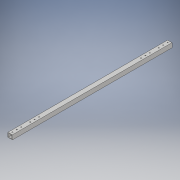
# Autodesk Inventor part: 3ft 1x1
Saved by Autodesk Inventor 2018 (Build 220112000, 112)
## iProperties
Created: 2018-12-30
Part Number: 3ft 1x1
Material: Generic
Document SubType Name: Modeling
Designer: maste
Density: 1 g/cm^3
Appearance: Default
Author: maste
Autodesk Inventor part; units mm, degrees
ref_plane "YZ Plane" through (0, 0, 0) normal (1, 0, 0) x (0, 1, 0)
ref_plane "XZ Plane" through (0, 0, 0) normal (0, 1, 0) x (-1, 0, 0)
ref_plane "XY Plane" through (0, 0, 0) normal (0, 0, 1) x (1, 0, 0)
sketch "Sketch1" plane through (0, 0, 0) normal (0, 0, 1) x (1, 0, 0)
  line L0 (0, 0) -> (25.4, 0)
  line L1 (25.4, 0) -> (25.4, 25.4)
  line L2 (25.4, 25.4) -> (0, 25.4)
  line L3 (0, 25.4) -> (0, 0)
  line L4 (3.175, 22.225) -> (22.225, 22.225)
  line L5 (22.225, 22.225) -> (22.225, 3.175)
  line L6 (22.225, 3.175) -> (3.175, 3.175)
  line L7 (3.175, 3.175) -> (3.175, 22.225)
  dimension "d0" = 25.4
  dimension "d1" = 25.4
  dimension "d2" = 3.175
  constraints: 16 end point, 4 parallel, 2 perpendicular, 1 horizontal, 3 other
  measures "d0" distance of L2.end L1.end
  measures "d1" distance of L1.end L0.end
  measures "d2" distance between parallel lines of L2 L4
extrude "Extrusion1" add sketch "Sketch1" along normal blind 914.4
sketch "Sketch2" plane through (0, 25.4, 0) normal (0, 1, 0) x (1, 0, 0)
  line L0 (0, 0) -> (25.4, 0) construction
  line L1 (12.7, 0) -> (12.7, -12.7) construction
  line L2 (12.7, -12.7) -> (12.7, -38.1) construction
  line L3 (12.7, -38.1) -> (12.7, -63.5) construction
  line L4 (0, 0) -> (0, -914.4) construction
  line L5 (0, 0) -> (0, -139.7) construction
  line L6 (0, -139.7) -> (25.4, -139.7) construction
  line L7 (12.7, -139.7) -> (12.7, -114.3) construction
  line L8 (12.7, -114.3) -> (12.7, -165.1) construction
  line L9 (0, -457.2) -> (25.4, -457.2) construction
  line L10 (25.4, 0) -> (25.4, -914.4) construction
  circle A0 centre (12.7, -139.7) radius 2.5797
  circle A1 centre (12.7, -114.3) radius 2.5797
  circle A2 centre (12.7, -165.1) radius 2.5797
  circle A3 centre (12.7, -63.5) radius 2.5797
  circle A4 centre (12.7, -38.1) radius 2.5797
  circle A5 centre (12.7, -12.7) radius 2.5797
  circle A6 centre (12.7, -774.7) radius 2.5797
  circle A7 centre (12.7, -800.1) radius 2.5797
  circle A8 centre (12.7, -749.3) radius 2.5797
  circle A9 centre (12.7, -850.9) radius 2.5797
  circle A10 centre (12.7, -876.3) radius 2.5797
  circle A11 centre (12.7, -901.7) radius 2.5797
  dimension "d5" = 12.7
  dimension "d6" = 25.4
  dimension "d7" = 25.4
  dimension "d8" = 139.7
  dimension "d9" = 25.4
  dimension "d10" = 50.8
  dimension "d11" = 5.1594
  constraints: 16 end point, 12 centre point, 6 coincident, 6 symmetric about line, 4 midpoint, 4 point on line, 2 vertical, 1 perpendicular, 6 other
  measures "d5" distance of L1.start L1.end
  measures "d6" distance of L1.end L2.end
  measures "d7" distance of L2.end L3.end
  measures "d8" distance of L0.start L5.end
  measures "d9" distance of L7.start L7.end
  measures "d10" distance of L7.end L8.end
  measures "d11" diameter of A0
extrude "Extrusion2" cut sketch "Sketch2" against normal blind 914.4
body "Solid1"
